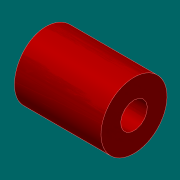
# Autodesk Inventor part: A1-19027-400-13 HCWI plug
Saved by Autodesk Inventor 2017.3 (Build 213257000, 257)
## iProperties
Created: 2019-08-16
Part Number: A1-19027-400-13 HCWI plug
Material: Iron, HCWI
Document SubType Name: Modeling
Designer: GVD
Density: 7.33517 g/cm^3
Appearance: Iron Gray(1)
Mass: 1571.47 g
Surface Area: 250.388 cm^2
Volume: 214.237 cm^3
Description: Ø2 1/2" x 3 5/16" HCWI PLUG, ASTM A532 CLASS III TYPE A, PF#(TBD)
Author: GVD
Autodesk Inventor part; units mm, degrees
ref_plane "YZ Plane" through (0, 0, 0) normal (1, 0, 0) x (0, 1, 0)
ref_plane "XZ Plane" through (0, 0, 0) normal (0, 1, 0) x (-1, 0, 0)
ref_plane "XY Plane" through (0, 0, 0) normal (0, 0, 1) x (1, 0, 0)
sketch "Sketch1" plane through (0, 0, 0) normal (0, 0, 1) x (1, 0, 0)
  line L0 (0, 0) -> (444.5, 0)
  line L1 (0, 0) -> (0, 31.5)
  line L2 (0, 31.5) -> (444.5, 31.5)
  line L3 (444.5, 31.5) -> (444.5, 12.7)
  line L4 (444.5, 12.7) -> (393.7, 12.7)
  line L5 (393.7, 12.7) -> (393.7, 0)
  dimension "d0" = 444.5
  dimension "d1" = 63
  dimension "d2" = 25.4
  dimension "d4" = 50.8
  constraints: 12 end point, 4 perpendicular, 2 point on line, 1 horizontal, 1 vertical
  measures "d0" distance of L0.start L0.end
  measures "d1" diameter of L2 L0
  measures "d2" diameter of L4 L0
  measures "d4" distance between parallel lines of L3 L5
revolve "Revolution1" add sketch "Sketch1" angle 360 about axis through (0, 0, 0) along (1, 0, 0)
fillet "Fillet1" radius 1.5875 1 edges at (393.7, -12.7, 0)
sketch "Sketch2" plane through (0, 0, 0) normal (0, 0, 1) x (1, 0, 0)
  circle A0 centre (0, 0) radius 361.95
  dimension "d9" = 723.9
  constraints: 1 centre point, 1 coincident
  measures "d9" diameter of A0
extrude "Extrusion1" cut sketch "Sketch2" along normal through all both and the other way through all
body "Solid1"
